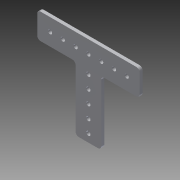
# Autodesk Inventor part: Roller Crossbar Gusset (Custom)
Saved by Autodesk Inventor 2014 (Build 180170000, 170)
## iProperties
Created: 2014-01-20
Part Number: Roller Crossbar Gusset (Custom)
Material: Aluminum 6061
Document SubType Name: Modeling
Designer: Michael
Density: 2.71 g/cm^3
Appearance: Aluminum - Flat
Author: Michael
Autodesk Inventor part; units mm, degrees
ref_plane "YZ Plane" through (0, 0, 0) normal (1, 0, 0) x (0, 1, 0)
ref_plane "XZ Plane" through (0, 0, 0) normal (0, 1, 0) x (-1, 0, 0)
ref_plane "XY Plane" through (0, 0, 0) normal (0, 0, 1) x (1, 0, 0)
sketch "Sketch1" plane through (0, 0, 0) normal (0, 0, 1) x (1, 0, 0)
  line L0 (0, 0) -> (101.6, 0)
  line L1 (101.6, 0) -> (101.6, -25.4)
  line L2 (101.6, -25.4) -> (63.5, -25.4)
  line L3 (63.5, -25.4) -> (63.5, -88.9)
  line L4 (63.5, -88.9) -> (38.1, -88.9)
  line L5 (38.1, -88.9) -> (38.1, -25.4)
  line L6 (38.1, -25.4) -> (0, -25.4)
  line L7 (0, -25.4) -> (0, 0)
  circle A0 centre (12.7, -12.7) radius 2.0701
  circle A1 centre (25.4, -12.7) radius 2.0701
  circle A2 centre (38.1, -12.7) radius 2.0701
  circle A3 centre (50.8, -12.7) radius 2.0701
  circle A4 centre (50.8, -30.1625) radius 2.0701
  circle A5 centre (50.8, -42.8625) radius 2.0701
  circle A6 centre (50.8, -55.5625) radius 2.0701
  circle A7 centre (50.8, -68.2625) radius 2.0701
  circle A8 centre (50.8, -80.9625) radius 2.0701
  circle A9 centre (63.5, -12.7) radius 2.0701
  circle A10 centre (76.2, -12.7) radius 2.0701
  circle A11 centre (88.9, -12.7) radius 2.0701
  dimension "d0" = 101.6
  dimension "d1" = 25.4
  dimension "d2" = 38.1
  dimension "d3" = 25.4
  dimension "d4" = 88.9
  dimension "d5" = 4.1402
  dimension "d6" = 12.7
  dimension "d7" = 12.7
  dimension "d10" = 12.7
  dimension "d15" = 4.7625
  dimension "d18" = 12.7
  dimension "d23" = 12.7
  constraints: 16 end point, 12 centre point, 7 parallel, 2 horizontal, 1 equal radius, 1 perpendicular, 1 vertical, 20 other
  measures "d0" distance of L0.start L0.end
  measures "d1" distance of L0.end L1.end
  measures "d2" distance of L1.end L2.end
  measures "d3" distance of L3.end L4.end
  measures "d4" distance between parallel lines of L0 L4
  measures "d5" diameter of A0
  measures "d6" distance from line of L6 A0.centre
  measures "d7" distance from line of L7 A0.centre
  measures "d10" distance of A0.centre A1.centre
  measures "d15" distance from line of L2 A4.centre
  measures "d18" distance of A4.centre A5.centre
  measures "d23" distance from line of L5 A4.centre
extrude "Extrusion1" add sketch "Sketch1" along normal blind 3.175
fillet "Fillet1" radius 3.175 8 edges at (63.5, -25.4, 1.5875) (101.6, -25.4, 1.5875) (101.6, 0, 1.5875) (0, 0, 1.5875) (0, -25.4, 1.5875) (38.1, -25.4, 1.5875) (38.1, -88.9, 1.5875) (63.5, -88.9, 1.5875)
body "Solid1"
